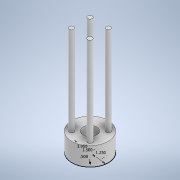
# Autodesk Inventor part: Chamber Top
Saved by Autodesk Inventor 2022 (Build 260153000, 153)
## iProperties
Created: 2022-04-18
Part Number: Chamber Top
Material: Generic
Document SubType Name: Modeling
Designer: tgr41
Density: 1 g/cm^3
Appearance: Default
Author: tgr41
Autodesk Inventor part; units mm, degrees
ref_plane "YZ Plane" through (0, 0, 0) normal (1, 0, 0) x (0, 1, 0)
ref_plane "XZ Plane" through (0, 0, 0) normal (0, 1, 0) x (-1, 0, 0)
ref_plane "XY Plane" through (0, 0, 0) normal (0, 0, 1) x (1, 0, 0)
sketch "Sketch1" plane through (0, 0, 0) normal (0, 1, 0) x (-1, 0, 0)
  circle A0 centre (0, 0) radius 50.165
  circle A1 centre (0, 0) radius 19.05
  line L0 (0, 50.165) -> (0, -50.165)
  line L1 (50.165, 0) -> (-50.165, 0)
  line L2 (0, 0) -> (-31.75, 0)
  line L3 (0, 0) -> (-25.4, 0)
  line L4 (0, 25.4) -> (0, 0)
  circle A2 centre (-25.4, 25.4) radius 6.35
  circle A3 centre (25.4, 25.4) radius 6.35
  circle A4 centre (-25.4, -25.4) radius 6.35
  circle A5 centre (25.4, -25.4) radius 6.35
  dimension "d0" = 100.33
  dimension "d1" = 38.1
  dimension "d6" = 31.75
  dimension "d10" = 12.7
  constraints: 10 end point, 6 centre point, 4 point on circle, 3 symmetric about line, 2 coincident, 2 horizontal, 1 point on line, 1 vertical, 3 other
  measures "d0" diameter of A0
  measures "d1" diameter of A1
  measures "d6" distance of L2.start L2.end
  measures "d10" diameter of A2
extrude "Extrusion1" add sketch "Sketch1" along normal blind 50.8 contours L1 A1 L0 A0 | A0 L0 A1 L1 | L0 A1 L1 A0 | A0 L1 A1 L0 | L1 L0 A1 | A1 L0 L1 | A1 L1 L0 | L0 L1 A1 | A2 | A3 | A4 | A5
extrude "Extrusion2" cut sketch "Sketch1" along normal blind 285.242 contours L1 L0 A1 | A1 L0 L1 | A1 L1 L0 | L0 L1 A1
extrude "Extrusion3" add sketch "Sketch1" along normal blind 297.561 contours A2 | A3 | A4 | A5
body "Solid1"
